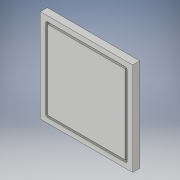
# Autodesk Inventor part: cy oring
Saved by Autodesk Inventor 2018 (Build 220112000, 112)
## iProperties
Created: 2018-10-17
Part Number: cy oring
Material: Generic
Document SubType Name: Modeling
Designer: STS
Density: 1 g/cm^3
Appearance: Default
Author: STS
Autodesk Inventor part; units mm, degrees
ref_plane "YZ Plane" through (0, 0, 0) normal (1, 0, 0) x (0, 1, 0)
ref_plane "XZ Plane" through (0, 0, 0) normal (0, 1, 0) x (-1, 0, 0)
ref_plane "XY Plane" through (0, 0, 0) normal (0, 0, 1) x (1, 0, 0)
sketch "Sketch1" plane through (0, 0, 0) normal (0, 0, 1) x (1, 0, 0)
  line L0 (64.262, -65.278) -> (-64.262, -65.278)
  line L1 (-64.262, -65.278) -> (-64.262, 65.278)
  line L2 (-64.262, 65.278) -> (64.262, 65.278)
  line L3 (64.262, 65.278) -> (64.262, -65.278)
  line L4 (76.454, -76.962) -> (-76.454, -76.962)
  line L5 (-76.454, -76.962) -> (-76.454, 76.962)
  line L6 (-76.454, 76.962) -> (76.454, 76.962)
  line L7 (76.454, 76.962) -> (76.454, -76.962)
  line L8 (64.262, 68.453) -> (-64.262, 68.453)
  line L9 (-67.437, 65.278) -> (-67.437, -65.278)
  line L10 (-64.262, -68.453) -> (64.262, -68.453)
  line L11 (67.437, -65.278) -> (67.437, 65.278)
  arc A0 (-64.262, 68.453) -> (-67.437, 65.278) centre (-64.262, 65.278) ccw
  arc A1 (67.437, 65.278) -> (64.262, 68.453) centre (64.262, 65.278) ccw
  arc A2 (64.262, -68.453) -> (67.437, -65.278) centre (64.262, -65.278) ccw
  arc A3 (-67.437, -65.278) -> (-64.262, -68.453) centre (-64.262, -65.278) ccw
  point P0 (0, 0)
  dimension "d0" = 128.524
  dimension "d1" = 130.556
  dimension "d2" = 152.908
  dimension "d3" = 153.924
  dimension "d4" = 3.175
  dimension "d5" = 3.175
  constraints: 24 end point, 8 point on circle, 8 tangent, 6 parallel, 4 centre point, 3 equal radius, 3 perpendicular, 2 horizontal, 3 other
  measures "d0" distance of L1.end L2.end
  measures "d1" distance of L0.end L1.end
  measures "d2" distance of L5.end L6.end
  measures "d3" distance of L4.end L5.end
  measures "d4" distance between parallel lines of L2 L8
  measures "d5" radius of A0
extrude "Extrusion1" add sketch "Sketch1" against normal blind 11.6586
body "Solid1"
